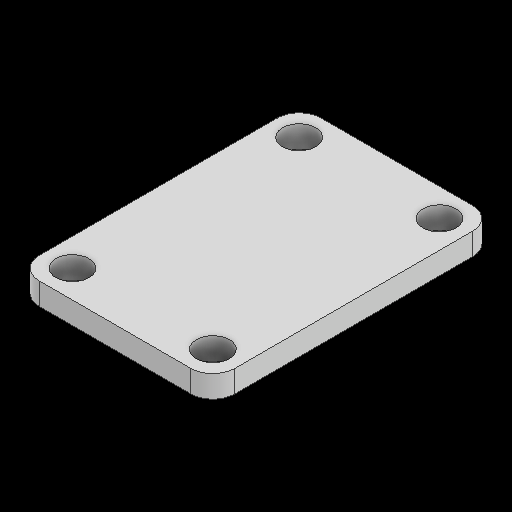
# Autodesk Inventor part: Temp_Basis_Platte
Saved by Autodesk Inventor 2027.1 (Build 311270010, 270A)
## iProperties
Created: 2026-10-08
Part Number: Temp_Basis_Platte
Material: Generisch
Document SubType Name: Modeling
Designer: josia
Density: 1 g/cm^3
Appearance: Vorgabe
Author: josia
Autodesk Inventor part; units mm, degrees
ref_plane "YZ Plane" through (0, 0, 0) normal (1, 0, 0) x (0, 1, 0)
ref_plane "XZ Plane" through (0, 0, 0) normal (0, 1, 0) x (-1, 0, 0)
ref_plane "XY Plane" through (0, 0, 0) normal (0, 0, 1) x (1, 0, 0)
sketch "Skizze1" plane through (0, 0, 0) normal (0, 1, 0) x (-1, 0, 0)
  line L0 (-8.85, -12.75) -> (8.85, -12.75)
  line L1 (8.85, -12.75) -> (8.85, 12.75)
  line L2 (8.85, 12.75) -> (-8.85, 12.75)
  line L3 (-8.85, 12.75) -> (-8.85, -12.75)
  line L4 (-8.85, -12.75) -> (8.85, 12.75) construction
  line L5 (8.85, -12.75) -> (-8.85, 12.75) construction
  point P0 (0, 0)
  dimension "d0" = 17.7
  dimension "d1" = 25.5
  constraints: 12 end point, 2 midpoint, 2 parallel, 1 horizontal, 1 perpendicular
  measures "d0" distance of L2.end L1.end
  measures "d1" distance of L1.end L0.end
extrude "Extrusion1" add sketch "Skizze1" along normal blind 2
fillet "Rundung1" radius 2 4 edges at (-8.85, 1, 12.75) (8.85, 1, 12.75) (8.85, 1, -12.75) (-8.85, 1, -12.75)
sketch "Skizze3" plane through (0, 2, 0) normal (0, 1, 0) x (1, 0, 0)
  line L0 (6.35, 10.25) -> (-6.35, 10.25)
  line L1 (-6.35, 10.25) -> (-6.35, -10.25)
  line L2 (-6.35, -10.25) -> (6.35, -10.25)
  line L3 (6.35, -10.25) -> (6.35, 10.25)
  line L4 (6.35, 10.25) -> (-6.35, -10.25) construction
  line L5 (-6.35, 10.25) -> (6.35, -10.25) construction
  line L6 (6.85, 12.75) -> (-6.85, 12.75) projected
  line L7 (-8.85, 10.75) -> (-8.85, -10.75) projected
  circle A0 centre (-6.35, 10.25) radius 1.5
  circle A1 centre (6.35, 10.25) radius 1.5
  circle A2 centre (6.35, -10.25) radius 1.5
  circle A3 centre (-6.35, -10.25) radius 1.5
  point P0 (0, 0)
  dimension "d16" = 2.5
  dimension "d17" = 2.5
  dimension "d18" = 3
  dimension "d19" = 3
  dimension "d20" = 3
  dimension "d21" = 3
  constraints: 12 end point, 4 centre point, 4 coincident, 2 midpoint, 2 parallel, 1 horizontal, 1 perpendicular
  measures "d16" distance between parallel lines of L7 L1
  measures "d17" distance between parallel lines of L6 L0
  measures "d18" diameter of A0
  measures "d19" diameter of A1
  measures "d20" diameter of A2
  measures "d21" diameter of A3
extrude "Extrusion2" cut sketch "Skizze3" against normal blind 3 contours A0 L1 L0 | L0 L1 A0 | A1 L3 L0 | L0 L3 A1 | A3 L2 L1 | L1 L2 A3 | A2 L2 L3 | L3 L2 A2
equation "\"d22\" = d21"
